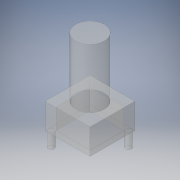
# Autodesk Inventor part: VLP-350-F
Saved by Autodesk Inventor 2016 (Build 200138000, 138)
## iProperties
Created: 2015-10-20
Part Number: VLP-350-F
Material: Polycarbonate, Clear
Document SubType Name: Modeling
Designer: jeremyhale
Density: 1.2 g/cm^3
Appearance: Polycarbonate - Clear
Author: jeremyhale
Autodesk Inventor part; units mm, degrees
ref_plane "YZ Plane" through (0, 0, 0) normal (1, 0, 0) x (0, 1, 0)
ref_plane "XZ Plane" through (0, 0, 0) normal (0, 1, 0) x (-1, 0, 0)
ref_plane "XY Plane" through (0, 0, 0) normal (0, 0, 1) x (1, 0, 0)
sketch "Sketch1" plane through (0, 0, 0) normal (0, 1, 0) x (-1, 0, 0)
  line L0 (-2.3495, 2.3495) -> (2.3495, 2.3495)
  line L1 (2.3495, 2.3495) -> (2.3495, -2.3495)
  line L2 (2.3495, -2.3495) -> (-2.3495, -2.3495)
  line L3 (-2.3495, -2.3495) -> (-2.3495, 2.3495)
  line L4 (-2.3495, 2.3495) -> (2.3495, -2.3495) construction
  line L5 (2.3495, 2.3495) -> (-2.3495, -2.3495) construction
  point P0 (0, 0)
  dimension "d0" = 4.699
  dimension "width" = 4.699
  constraints: 12 end point, 2 midpoint, 2 parallel, 1 horizontal, 1 perpendicular
  measures "d0" distance of L1.end L2.end
  measures "width" distance of L0.end L1.end
extrude "Extrusion1" add sketch "Sketch1" along normal blind 2.667
sketch "Sketch2" plane through (0, 2.667, 0) normal (0, 1, 0) x (1, 0, 0)
  circle A0 centre (0, 0) radius 1.4986
  dimension "d4" = 2.9972
  constraints: 1 centre point, 1 coincident
  measures "d4" diameter of A0
extrude "Extrusion2" add sketch "Sketch2" along normal blind 6.223
sketch "Sketch3" plane through (0, 0, 0) normal (0, -1, 0) x (1, 0, 0)
  line L0 (-1.778, 1.778) -> (1.778, 1.778)
  line L1 (1.778, 1.778) -> (1.778, -1.778)
  line L2 (1.778, -1.778) -> (-1.778, -1.778)
  line L3 (-1.778, -1.778) -> (-1.778, 1.778)
  line L4 (-1.778, 1.778) -> (1.778, -1.778) construction
  line L5 (1.778, 1.778) -> (-1.778, -1.778) construction
  point P0 (0, 0)
  dimension "d7" = 3.556
  dimension "d8" = 3.556
  constraints: 12 end point, 2 midpoint, 2 parallel, 1 horizontal, 1 perpendicular
  measures "d7" distance of L1.end L2.end
  measures "d8" distance of L0.end L1.end
extrude "Extrusion3" cut sketch "Sketch3" against normal blind 2.159
sketch "Sketch4" plane through (0, 0, 0) normal (0, -1, 0) x (1, 0, 0)
  circle A0 centre (-2.032, 2.032) radius 0.2921
  circle A1 centre (2.032, -2.032) radius 0.2921
  point P0 (0, 0)
  point P1 (0, 0)
  dimension "d11" = 0.5842
  dimension "d12" = 2.032
  dimension "d13" = 2.032
  dimension "d16" = 360
  constraints: 2 centre point, 1 coincident, 5 other
  measures "d11" diameter of A0
  measures "d12" horizontal distance of point (0, 0) A0.centre
  measures "d13" horizontal distance of point (0, 0) A0.centre
extrude "Extrusion4" add sketch "Sketch4" along normal blind 1.524
equation "\"d0\" = width"
body "Solid1"
